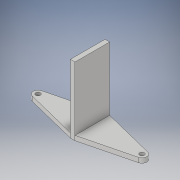
# Autodesk Inventor part: крепление
Saved by Autodesk Inventor 2019 (Build 230136000, 136)
## iProperties
Created: 2019-10-05
Part Number: крепление
Material: Типовые
Document SubType Name: Modeling
Designer: Iliga
Density: 1 g/cm^3
Appearance: По умолчанию
Author: Iliga
Autodesk Inventor part; units mm, degrees
ref_plane "YZ Plane" through (0, 0, 0) normal (1, 0, 0) x (0, 1, 0)
ref_plane "XZ Plane" through (0, 0, 0) normal (0, 1, 0) x (-1, 0, 0)
ref_plane "XY Plane" through (0, 0, 0) normal (0, 0, 1) x (1, 0, 0)
sketch "Эскиз1" plane through (0, 0, 0) normal (0, 1, 0) x (-1, 0, 0)
  circle A0 centre (45, 0) radius 2
  line L0 (-2, 15) -> (2, 15)
  line L1 (2, 15) -> (2, -15)
  line L2 (2, -15) -> (-2, -15)
  line L3 (-2, -15) -> (-2, 15)
  line L4 (-2, 15) -> (2, -15) construction
  line L5 (2, 15) -> (-2, -15) construction
  arc A1 (46, -4) -> (46, 4) centre (45, 0) ccw
  line L6 (2, 15) -> (46, 4)
  line L7 (46, -4) -> (2, -15)
  line L8 (0, 18) -> (0, -15) construction
  circle A2 centre (-45, 0) radius 2
  arc A3 (-46, 4) -> (-46, -4) centre (-45, 0) ccw
  line L9 (-2, 15) -> (-46, 4)
  line L10 (-46, -4) -> (-2, -15)
  point P0 (0, 0)
  point P1 (0, 0)
  dimension "d0" = 4
  dimension "d19" = 4
  dimension "d20" = 45
  dimension "d21" = 30
  dimension "d22" = 4
  constraints: 22 end point, 4 centre point, 4 point on circle, 4 symmetric about line, 3 coincident, 3 midpoint, 2 parallel, 2 tangent, 1 horizontal, 1 horizontal alignment, 1 perpendicular, 1 vertical alignment, 2 other
  measures "d0" diameter of A0
  measures "d19" distance between parallel lines of L1 L3
  measures "d20" distance of point (0, 0) A0.centre
  measures "d21" distance between parallel lines of L2 L0
  measures "d22" vertical distance of A0.centre L7.start
extrude "Выдавливание2" add sketch "Эскиз1" along normal blind 4 contours L3 L10 A3 L9 | L6 A1 L7 L1
extrude "Выдавливание3" add sketch "Эскиз1" along normal blind 59 contours L0 L1 L2 L3
